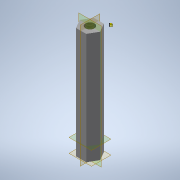
# Autodesk Inventor part: Steun stuk
Saved by Autodesk Inventor 2021 (Build 250183000, 183)
## iProperties
Manager: PJ / DCS
Company: Emmaüs Bovenbouw Aalter
Created: 2020-11-06
Part Number: Steun stuk
Material: S235
Catalog Web Link: http://emmausbovenbouw.op-weg.be/
Vendor: Emmaüsinstituut Bovenbouw Aalter
Document SubType Name: Modeling
Designer: Antho
Engineer: Declercq St.
Manufacturer: Standard
Standards Organization: Custom
Density: 7.86 g/cm^3
Appearance: Steel
Title: Algemene titel
Subject: Specifieke titel
Author: Antho
Keywords: Ruwe Ø xxxxx
Comments: Opmerking
Autodesk Inventor part; units mm, degrees
sketch "Sketch1" plane through (0, 0, 0) normal (0, 0, 1) x (1, 0, 0)
  line L0 (0, 2.8582) -> (0, -2.8582) construction
  line L1 (-5.7775, 0) -> (5.7775, 0) construction
  line L2 (0, 0) -> (4, 0)
  line L3 (4, 0) -> (-4, 0)
  circle A0 centre (0, 0) radius 4
  line L4 (0, 0) -> (-2, 3.4641)
  line L5 (0, 0) -> (4, 0) construction
  line L6 (0, 0) -> (2, 3.4641)
  line L7 (0, 0) -> (4, 0) construction
  line L8 (0, 0) -> (4, 0)
  line L9 (0, 0) -> (2, -3.4641)
  line L10 (0, 0) -> (-2, -3.4641)
  line L11 (-2, 3.4641) -> (2, 3.4641)
  line L12 (2, 3.4641) -> (4, 0)
  line L13 (4, 0) -> (2, -3.4641)
  line L14 (2, -3.4641) -> (-2, -3.4641)
  line L15 (-2, -3.4641) -> (-4, 0)
  line L16 (-4, 0) -> (-2, 3.4641)
  dimension "d1" = 4
  dimension "d2" = 8
  dimension "d3" = 120
  dimension "d4" = 60
  constraints: 34 end point, 5 point on circle, 4 equal length, 3 coincident, 3 horizontal, 3 point on line, 2 midpoint, 1 centre point, 1 vertical
  measures "d1" distance of L2.start L2.end
  measures "d2" distance of L2.end L3.end
  measures "d3" angle of L5 L4
  measures "d4" angle of L7 L6
extrude "Extrusion1" add sketch "Sketch1" along normal blind 43.5 contours L6 L12 L2 | L10 L15 L3 | L3 L16 L4 | L4 L11 L6 | L2 L13 L9 | L9 L14 L10
sketch "Sketch5" plane through (0, 0, 43.5) normal (0, 0, 1) x (1, 0, 0)
  point P0 (0, 0)
  point P1 (0, 0)
  constraints: 1 coincident
hole "Hole2" at (0, 0, 43.5) direction (0, 0, -1) diameter 3.4587 depth 8 thread size "M4x0.5" class "6H" standard "ISO Metric profile"
sketch "Sketch6" plane through (0, 0, 0) normal (0, 0, -1) x (-1, 0, 0)
  point P0 (0, 0)
  point P1 (0, 0)
  constraints: 1 coincident
hole "Hole3" at (0, 0, 0) direction (0, 0, 1) diameter 3.4587 depth 10.8 thread size "M4x0.5" class "6H" standard "ISO Metric profile"
ref_plane "Work Plane1" through (0, 0, 5.4) normal (0, 0, -1) x (-1, 0, 0)
body "Solid1"
